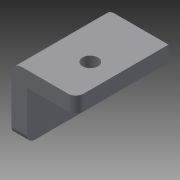
# Autodesk Inventor part: EE_adapter_forOld
Saved by Autodesk Inventor 2015 (Build 190159000, 159)
## iProperties
Created: 2014-12-11
Part Number: EE_adapter_forOld
Material: Generic
Document SubType Name: Modeling
Designer: rawrdong
Density: 1 g/cm^3
Appearance: Default
Author: rawrdong
Autodesk Inventor part; units mm, degrees
ref_plane "YZ Plane" through (0, 0, 0) normal (1, 0, 0) x (0, 1, 0)
ref_plane "XZ Plane" through (0, 0, 0) normal (0, 1, 0) x (-1, 0, 0)
ref_plane "XY Plane" through (0, 0, 0) normal (0, 0, 1) x (1, 0, 0)
sketch "Sketch1" plane through (0, 0, 0) normal (0, 1, 0) x (-1, 0, 0)
  line L0 (0, -2) -> (0, -12.5)
  line L1 (0, -12.5) -> (-3, -12.5)
  line L2 (-2, 0) -> (-12.5, 0)
  line L3 (-12.5, 0) -> (-12.5, -3)
  line L4 (-12.5, -3) -> (-3.1, -3)
  line L5 (-3, -3.1) -> (-3, -12.5)
  line L6 (0, 0) -> (-12.1249, -12.1249) construction
  arc A0 (-3, -3.1) -> (-3.1, -3) centre (-3.1, -3.1) ccw
  arc A1 (0, -2) -> (-2, 0) centre (-2, -2) ccw
  line L7 (-15.0828, 0) -> (2.9971, 0) projected
  point P0 (-3, -3)
  dimension "d4" = 3
  dimension "d8" = 0.1
  dimension "d9" = 2
  dimension "d16" = 90
  dimension "d17" = 12.5
  constraints: 14 end point, 5 perpendicular, 5 point on line, 4 point on circle, 4 tangent, 2 centre point, 1 horizontal, 1 vertical
  measures "d4" distance of L2.end L3.end
  measures "d8" radius of A0
  measures "d9" radius of A1
  measures "d16" angle of L4 L5
  measures "d17" distance from line of L7 L0.end
extrude "Extrusion1" add sketch "Sketch1" along normal blind 15
sketch "Sketch2" plane through (0, 15, 0) normal (0, 1, 0) x (1, 0, 0)
  line L0 (0, 12.5) -> (0, 2) projected
  line L1 (2, 0) -> (12.5, 0) projected
  line L2 (12.5, 0) -> (12.5, 3) projected
  line L3 (12.5, 3) -> (3.1, 3) projected
  line L4 (3, 3.1) -> (3, 12.5) projected
  line L5 (3, 12.5) -> (0, 12.5) projected
  line L6 (12.5, 3) -> (3, 12.5)
  arc A0 (0, 2) -> (2, 0) centre (2, 2) ccw projected
  arc A1 (3, 3.1) -> (3.1, 3) centre (3.1, 3.1) ccw projected
  point P0 (0, 0)
  constraints: 2 end point
extrude "Extrusion2" add sketch "Sketch2" along normal blind 3
sketch "Sketch3" plane through (12.5, 0, -3) normal (0, 0, -1) x (-1, 0, 0)
  line L0 (0, 0) -> (9.4, 0) projected
  line L1 (0, 0) -> (0, 15) projected
  circle A0 centre (4.7, 7.5) radius 1.5
  line L2 (9.4, 0) -> (9.4, 15) projected
  line L3 (0, 15) -> (9.4, 15) projected
  point P0 (12.5, 0)
  point P1 (4.7, 0)
  point P2 (0, 7.5)
  dimension "d5" = 3
  constraints: 2 midpoint, 1 centre point, 1 horizontal alignment, 1 vertical alignment
  measures "d5" diameter of A0
extrude "Extrusion3" cut sketch "Sketch3" against normal through all contours A0
sketch "Sketch5" plane through (3, 0, -12.5) normal (1, 0, 0) x (0, 0, -1)
  circle A0 centre (-4.7, 7.5) radius 1.5
  line L0 (-9.4, 0) -> (0, 0) projected
  line L1 (0, 0) -> (0, 15) projected
  line L2 (-9.4, 15) -> (0, 15) projected
  line L3 (-9.4, 0) -> (-9.4, 15) projected
  point P0 (-12.5, 0)
  point P1 (-4.7, 0)
  point P2 (0, 7.5)
  dimension "d12" = 3
  constraints: 2 midpoint, 1 centre point, 1 horizontal alignment, 1 vertical alignment
  measures "d12" diameter of A0
extrude "Extrusion4" cut sketch "Sketch5" against normal through all contours A0
fillet "Fillet1" radius 1.5 2 edges at (1.5, 0, -12.5) (12.5, 0, -1.5)
body "Solid1"
